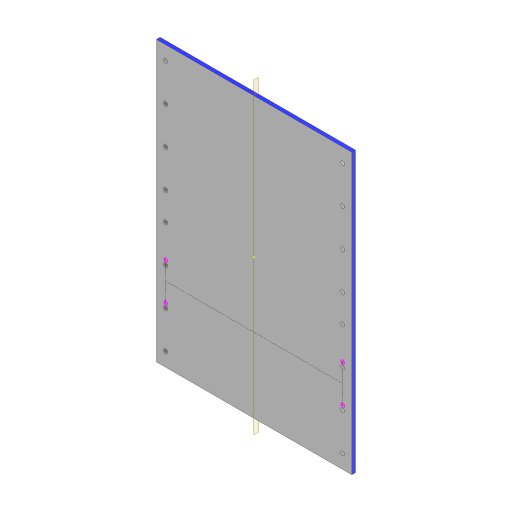
# Autodesk Inventor part: Передняя_Задняя фанера
Saved by Autodesk Inventor 2023.2 (Build 272271030, 271C)
## iProperties
Created: 2025-04-24
Part Number: Передняя_Задняя фанера
Material: Типовые
Document SubType Name: Modeling
Designer: Коноваленко
Density: 1 g/cm^3
Appearance: По умолчанию
Author: Коноваленко
Autodesk Inventor part; units mm, degrees
ref_plane "XZ Plane" through (0, 0, 0) normal (0, 1, 0) x (-1, 0, 0)
ref_plane "XY Plane" through (0, 0, 0) normal (0, 0, 1) x (1, 0, 0)
sketch "Эскиз1" plane through (0, 0, 0) normal (0, 0, 1) x (1, 0, 0)
  line L0 (-105, -150) -> (105, -150)
  line L1 (105, -150) -> (105, 150)
  line L2 (105, 150) -> (-105, 150)
  line L3 (-105, 150) -> (-105, -150)
  line L4 (-105, -150) -> (105, 150) construction
  line L5 (105, -150) -> (-105, 150) construction
  point P0 (0, 0)
  dimension "d0" = 300
  dimension "d1" = 210
  constraints: 12 end point, 2 midpoint, 2 parallel, 1 horizontal, 1 perpendicular
  measures "d0" distance of L2.end L0.start
  measures "d1" distance of L0.start L0.end
extrude "Выдавливание1" add sketch "Эскиз1" along normal mid plane 4
sketch "Эскиз2" plane through (0, 0, 2) normal (0, 0, 1) x (1, 0, 0)
  circle A0 centre (-95, 172.5) radius 2
  circle A1 centre (-95, 157.5) radius 2
  circle A2 centre (-95, 142.5) radius 2
  circle A3 centre (-95, 127.5) radius 2
  circle A4 centre (-95, 100) radius 2
  circle A5 centre (-95, 60) radius 2
  circle A6 centre (-95, 20) radius 2
  circle A7 centre (-95, -20) radius 2
  circle A8 centre (-95, -50) radius 2
  circle A9 centre (-95, -90) radius 2
  circle A10 centre (-95, -130) radius 2
  circle A11 centre (-95, -170) radius 2
  circle A12 centre (95, -170) radius 2
  circle A13 centre (95, -130) radius 2
  circle A14 centre (95, -90) radius 2
  circle A15 centre (95, -50) radius 2
  circle A16 centre (95, -20) radius 2
  circle A17 centre (95, 20) radius 2
  circle A18 centre (95, 60) radius 2
  circle A19 centre (95, 100) radius 2
  circle A20 centre (95, 127.5) radius 2
  circle A21 centre (95, 142.5) radius 2
  circle A22 centre (95, 157.5) radius 2
  circle A23 centre (95, 172.5) radius 2
  point P0 (0, 0)
  constraints: 24 centre point, 48 other
extrude "Выдавливание2" [suppressed]
sketch "Эскиз3" plane through (0, 0, -2) normal (0, 0, -1) x (-1, 0, 0)
  circle A0 centre (-95, 135) radius 2
  circle A1 centre (-95, 95) radius 2
  circle A2 centre (-95, 55) radius 2
  circle A3 centre (-95, 15) radius 2
  circle A4 centre (-95, -15) radius 2
  circle A5 centre (-95, -55) radius 2
  circle A6 centre (-95, -95) radius 2
  circle A7 centre (-95, -135) radius 2
  circle A8 centre (95, 135) radius 2
  circle A9 centre (95, 95) radius 2
  circle A10 centre (95, 55) radius 2
  circle A11 centre (95, 15) radius 2
  circle A12 centre (95, -55) radius 2
  circle A13 centre (95, -95) radius 2
  circle A14 centre (95, -135) radius 2
  circle A15 centre (95, -15) radius 2
  point P0 (0, 0)
  constraints: 16 centre point, 32 other
extrude "Выдавливание3" cut sketch "Эскиз3" against normal up to surface (4 mm away)
sketch "Эскиз4" plane through (0, 0, 2) normal (0, 0, 1) x (1, 0, 0)
  circle A0 centre (-95, -130) radius 2 projected
  circle A1 centre (95, -130) radius 2 projected
  line L0 (-95, -130) -> (95, -130) construction
  circle A2 centre (0, -130) radius 9.6845
  point P0 (0, 0)
  point P1 (0, -130)
  dimension "d8" = 19.369
  constraints: 2 end point, 1 centre point, 1 coincident, 1 horizontal, 1 midpoint
  measures "d8" diameter of A2
extrude "Выдавливание4" [suppressed]
sketch "Эскиз5" plane through (0, 0, 2) normal (0, 0, 1) x (1, 0, 0)
  circle A0 centre (-95, -90) radius 2 projected
  circle A1 centre (-95, -50) radius 2 projected
  line L0 (-95, -90) -> (-95, -50) construction
  circle A2 centre (95, -50) radius 2 projected
  circle A3 centre (95, -90) radius 2 projected
  line L1 (95, -50) -> (95, -90) construction
  line L2 (-95, -70) -> (95, -70) construction
  point P0 (0, 0)
  constraints: 6 end point, 2 midpoint, 2 vertical
sketch "Эскиз8" plane through (0, 0, 2) normal (0, 0, 1) x (1, 0, 0)
  circle A0 centre (20.984, -61.504) radius 0.9099
  circle A1 centre (21.0274, -78.5002) radius 0.9099
  circle A2 centre (-20.98, -78.5791) radius 0.9099
  circle A3 centre (-21.0095, -61.5642) radius 0.9099
  arc A4 (3.6101, -79.169) -> (3.5899, -75.7917) centre (3.6136, -77.4802) ccw
  line L0 (3.6101, -79.169) -> (-3.6226, -79.169)
  arc A5 (-3.5744, -75.7917) -> (-3.6226, -79.169) centre (-3.5227, -77.4814) ccw
  line L1 (3.5899, -75.7917) -> (-3.5744, -75.7917)
  line L2 (0, 210) -> (0, -210) projected
  line L3 (31.5, -70) -> (-31.5, -70)
  arc A6 (3.5899, -64.2083) -> (5.3022, -62.5018) centre (3.6136, -62.5198) ccw
  arc A7 (-5.2132, -62.4995) -> (-3.5744, -64.2083) centre (-3.5227, -62.5186) ccw
  line L4 (3.5899, -64.2083) -> (-3.5744, -64.2083)
  line L5 (-5.2132, -62.5377) -> (-5.2132, -58.4787)
  line L6 (-5.2132, -58.4787) -> (5.3022, -58.4787)
  line L7 (5.3022, -58.4787) -> (5.3022, -62.5377)
  circle A8 centre (-13, -69.9999) radius 8
  circle A9 centre (13, -69.9999) radius 8
  point P0 (0, 0)
  point P1 (3.6101, -60.831)
  point P2 (-3.6226, -60.831)
  dimension "d12" = 4.059
  dimension "d13" = 10.5154
  constraints: 14 end point, 10 centre point, 10 point on circle, 6 symmetric about line, 3 horizontal, 2 perpendicular, 2 point on line, 1 parallel, 1 vertical, 24 other
  measures "d12" distance of L6.end L7.end
  measures "d13" distance of L5.end L6.end
extrude "Выдавливание5" [suppressed]
